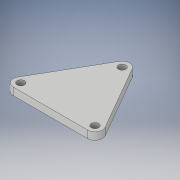
# Autodesk Inventor part: ternary_link
Saved by Autodesk Inventor 2019 (Build 230136000, 136)
## iProperties
Created: 2021-02-18
Part Number: ternary_link
Material: 一般
Document SubType Name: Modeling
Designer: wasd5
Density: 1 g/cm^3
Appearance: 預設
Author: wasd5
Autodesk Inventor part; units mm, degrees
ref_plane "YZ Plane" through (0, 0, 0) normal (1, 0, 0) x (0, 1, 0)
ref_plane "XZ Plane" through (0, 0, 0) normal (0, 1, 0) x (-1, 0, 0)
ref_plane "XY Plane" through (0, 0, 0) normal (0, 0, 1) x (1, 0, 0)
sketch "草圖1" plane through (0, 0, 0) normal (0, 1, 0) x (-1, 0, 0)
  line L0 (0, -57.735) -> (-50, 28.8675) construction
  line L1 (-50, 28.8675) -> (50, 28.8675) construction
  line L2 (50, 28.8675) -> (0, -57.735) construction
  arc A0 (-8.6603, -62.735) -> (8.6603, -62.735) centre (0, -57.735) ccw
  arc A1 (-50, 38.8675) -> (-58.6603, 23.8675) centre (-50, 28.8675) ccw
  arc A2 (58.6603, 23.8675) -> (50, 38.8675) centre (50, 28.8675) ccw
  line L3 (8.6603, -62.735) -> (58.6603, 23.8675)
  line L4 (-8.6603, -62.735) -> (-58.6603, 23.8675)
  line L5 (-50, 38.8675) -> (50, 38.8675)
  circle A3 centre (0, -57.735) radius 5
  circle A4 centre (50, 28.8675) radius 5
  circle A5 centre (-50, 28.8675) radius 5
  point P0 (0, 0)
  point P1 (0, 0)
  dimension "center_length" = 100
  dimension "d1" = 20
  dimension "hole" = 10
  constraints: 12 end point, 7 coincident, 6 centre point, 6 point on circle, 5 tangent, 4 equal radius, 2 horizontal, 7 other
  measures "center_length" distance of L0.start L0.end
  measures "d1" diameter of A0
  measures "hole" diameter of A3
extrude "擠出1" add sketch "草圖1" along normal blind 10
equation "\"d1\" = 2 * hole"
